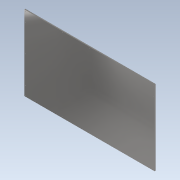
# Autodesk Inventor part: 101.001.01_Bodenplatte
Saved by Autodesk Inventor 2022 (Build 260153000, 153)
## iProperties
Created: 2021-11-25
Part Number: 101.001.01_Bodenplatte
Material: Stahl, hochfest, niedrig legiert
Document SubType Name: Modeling
Designer: Sebastian Seewald
Mass: 55577.7 g
Surface Area: 14517.6 cm^2
Volume: 7079.97 cm^3
Density: 7.85 g/cm^3
Appearance: Stahl - poliert
Author: Sebastian Seewald
Autodesk Inventor part; units mm, degrees
ref_plane "YZ Plane" through (0, 0, 0) normal (1, 0, 0) x (0, 1, 0)
ref_plane "XZ Plane" through (0, 0, 0) normal (0, 1, 0) x (-1, 0, 0)
ref_plane "XY Plane" through (0, 0, 0) normal (0, 0, 1) x (1, 0, 0)
sketch "Skizze1" plane through (0, 0, 0) normal (0, 0, 1) x (1, 0, 0)
  line L0 (2, 0) -> (1198, 0)
  line L1 (1200, 2) -> (1200, 688)
  line L2 (1198, 690) -> (2, 690)
  line L3 (0, 688) -> (0, 2)
  arc A0 (2, 690) -> (0, 688) centre (2, 688) ccw
  arc A1 (1200, 688) -> (1198, 690) centre (1198, 688) ccw
  arc A2 (1198, 0) -> (1200, 2) centre (1198, 2) ccw
  arc A3 (0, 2) -> (2, 0) centre (2, 2) ccw
  point P0 (0, 0)
  point P1 (1200, 690)
  point P2 (1200, 0)
  point P3 (0, 690)
  dimension "d0" = 1200
  dimension "d1" = 690
  dimension "d2" = 2
  constraints: 8 end point, 8 point on circle, 8 point on line, 8 tangent, 4 centre point, 3 equal radius, 2 parallel, 1 horizontal, 1 perpendicular
  measures "d0" distance of point (1200, 690) point (0, 690)
  measures "d1" distance of point (1200, 0) point (1200, 690)
  measures "d2" radius of A0
extrude "Extrusion1" add sketch "Skizze1" along normal blind 10
sketch "Sketch2" plane through (0, 0, 0) normal (0, 0, -1) x (-1, 0, 0)
  circle A0 centre (-10, 10) radius 3.25
  line L0 (-2, 0) -> (-1198, 0) projected
  line L1 (0, 688) -> (0, 2) projected
  line L2 (-600, -175.8373) -> (-600, 803.7474) construction
  line L3 (202.1324, 345) -> (-1409.3068, 345) construction
  circle A1 centre (-1190, 10) radius 3.25
  circle A2 centre (-10, 680) radius 3.25
  line L4 (-2, 690) -> (-1198, 690)
  circle A3 centre (-1190, 680) radius 3.25
  point P0 (0, 0)
  point P1 (-1200, 0)
  point P2 (-1200, 2)
  point P3 (0, 690)
  point P4 (-1200, 690)
  point P5 (-1200, 688)
  dimension "d5" = 6.5
  dimension "d6" = 10
  dimension "d7" = 10
  dimension "d8" = 600
  dimension "d9" = 345
  constraints: 10 symmetric about line, 6 end point, 4 centre point, 1 horizontal, 1 vertical, 3 other
  measures "d5" diameter of A0
  measures "d6" distance from line of L0 A0.centre
  measures "d7" distance from line of A0.centre L1
  measures "d8" distance between parallel lines of L1 L2
  measures "d9" distance between parallel lines of L0 L3
hole "Hole1" at (10, 10, 0) at (1190, 10, 0) at (1190, 680, 0) at (10, 680, 0) direction (0, 0, 1) diameter 6.5 end through all
sketch "Sketch3" plane through (0, 0, 0) normal (0, 0, -1) x (-1, 0, 0)
  circle A0 centre (-10, 590) radius 3
  line L0 (0, 688) -> (0, 2) projected
  line L1 (-1198, 690) -> (-2, 690) projected
  circle A1 centre (-10, 340) radius 3
  circle A2 centre (-10, 90) radius 3
  line L2 (-600, 869.8508) -> (-600, -209.8368) construction
  circle A3 centre (-1190, 590) radius 3
  circle A4 centre (-1190, 340) radius 3
  circle A5 centre (-1190, 90) radius 3
  circle A6 centre (-100, 680) radius 3
  circle A7 centre (-350, 680) radius 3
  circle A8 centre (-600, 680) radius 3
  circle A9 centre (-850, 680) radius 3
  circle A10 centre (-1100, 680) radius 3
  line L3 (113.1305, 345) -> (-1507.9608, 345) construction
  circle A11 centre (-100, 10) radius 3
  circle A12 centre (-350, 10) radius 3
  circle A13 centre (-600, 10) radius 3
  circle A14 centre (-850, 10) radius 3
  circle A15 centre (-1100, 10) radius 3
  point P0 (0, 0)
  dimension "d17" = 6
  dimension "d19" = 100
  dimension "d22" = 250
  dimension "d27" = 600
  dimension "d33" = 250
  dimension "d38" = 345
  constraints: 16 centre point, 8 symmetric about line, 4 end point, 2 horizontal, 2 vertical, 20 other
  measures "d17" diameter of A0
  measures "d19" distance from line of A0.centre L1
  measures "d22" distance of A0.centre A1.centre
  measures "d27" distance from line of L2 point (0, 0)
  measures "d33" distance of A6.centre A7.centre
  measures "d38" distance between parallel lines of L3 L1
hole "Hole2" at (10, 590, 0) at (10, 90, 0) at (100, 10, 0) at (350, 10, 0) at (600, 10, 0) at (600, 680, 0) at (850, 10, 0) at (1100, 10, 0) at (1190, 90, 0) at (1190, 340, 0) at (1190, 590, 0) at (1100, 680, 0) at (850, 680, 0) direction (0, 0, 1) diameter 6 end through all
sketch "Sketch4" plane through (0, 0, 0) normal (0, 0, -1) x (-1, 0, 0)
  circle A0 centre (-100, 680) radius 3
  line L0 (0, 688) -> (0, 2) projected
  line L1 (-1198, 690) -> (-2, 690) projected
  circle A1 centre (-350, 680) radius 3
  point P0 (0, 0)
  dimension "d46" = 100
  dimension "d47" = 10
  dimension "d48" = 6
  dimension "d51" = 250
  constraints: 2 centre point, 1 horizontal, 2 other
  measures "d46" distance from line of A0.centre L0
  measures "d47" distance from line of A0.centre L1
  measures "d48" diameter of A0
  measures "d51" distance of A0.centre A1.centre
hole "Hole3" at (100, 680, 0) direction (0, 0, 1) diameter 6 end through all
sketch "Sketch5" plane through (0, 0, 0) normal (0, 0, -1) x (-1, 0, 0)
  circle A0 centre (-350, 680) radius 3
  circle A1 centre (-100, 680) radius 3 projected
  line L0 (-1198, 690) -> (-2, 690) projected
  point P0 (0, 0)
  dimension "d63" = 250
  dimension "d64" = 10
  dimension "d65" = 6
  constraints: 1 centre point
  measures "d63" distance of A0.centre A1.centre
  measures "d64" distance from line of A0.centre L0
  measures "d65" diameter of A0
hole "Hole4" at (350, 680, 0) direction (0, 0, 1) diameter 6 end through all
sketch "Sketch6" plane through (0, 0, 0) normal (0, 0, -1) x (-1, 0, 0)
  circle A0 centre (-10, 340) radius 3
  circle A1 centre (-10, 590) radius 3 projected
  line L0 (0, 688) -> (0, 2) projected
  point P0 (0, 0)
  dimension "d73" = 250
  dimension "d74" = 10
  dimension "d75" = 6
  constraints: 1 centre point
  measures "d73" distance of A1.centre A0.centre
  measures "d74" distance from line of A0.centre L0
  measures "d75" diameter of A0
hole "Hole5" at (10, 340, 0) direction (0, 0, 1) diameter 6 end through all
equation "\"d10\" = d5"
equation "\"d39\" = d17"
equation "\"d56\" = d17"
equation "\"d66\" = d65"
equation "\"d76\" = d75"
